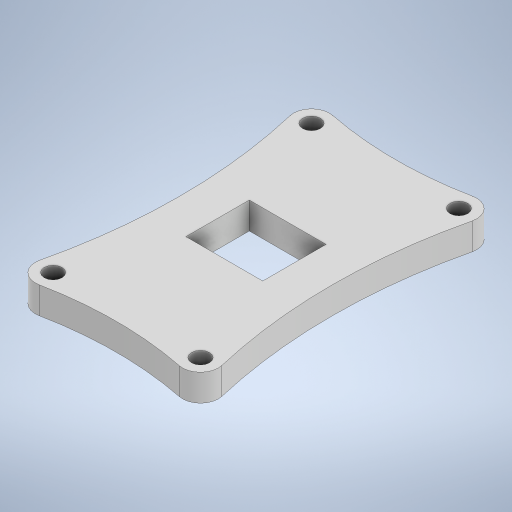
# Autodesk Inventor part: Seal_plate
Saved by Autodesk Inventor 2024.3 (Build 283343000, 343)
## iProperties
Created: 2024-11-18
Part Number: Seal_plate
Material: Generic
Document SubType Name: Modeling
Designer: magn1
Density: 1 g/cm^3
Appearance: Default
Author: magn1
Autodesk Inventor part; units mm, degrees
ref_plane "YZ Plane" through (0, 0, 0) normal (1, 0, 0) x (0, 1, 0)
ref_plane "XZ Plane" through (0, 0, 0) normal (0, 1, 0) x (-1, 0, 0)
ref_plane "XY Plane" through (0, 0, 0) normal (0, 0, 1) x (1, 0, 0)
sketch "Sketch1" plane through (0, 0, 0) normal (0, 1, 0) x (-1, 0, 0)
  line L0 (-8.25, 14.464) -> (8.25, 14.464) construction
  line L1 (8.25, 14.464) -> (8.25, -14.464) construction
  line L2 (8.25, -14.464) -> (-8.25, -14.464) construction
  line L3 (-8.25, -14.464) -> (-8.25, 14.464) construction
  line L4 (-8.25, 14.464) -> (8.25, -14.464) construction
  line L5 (8.25, 14.464) -> (-8.25, -14.464) construction
  circle A0 centre (8.25, 14.464) radius 1
  circle A1 centre (8.25, -14.464) radius 1
  circle A2 centre (-8.25, -14.464) radius 1
  circle A3 centre (-8.25, 14.464) radius 1
  line L6 (-4.3, 3.55) -> (4.3, 3.55)
  line L7 (4.3, 3.55) -> (4.3, -3.55)
  line L8 (4.3, -3.55) -> (-4.3, -3.55)
  line L9 (-4.3, -3.55) -> (-4.3, 3.55)
  line L10 (-4.3, 3.55) -> (4.3, -3.55) construction
  line L11 (4.3, 3.55) -> (-4.3, -3.55) construction
  circle A4 centre (8.25, 14.464) radius 2
  circle A5 centre (8.25, -14.464) radius 2
  circle A6 centre (-8.25, -14.464) radius 2
  circle A7 centre (-8.25, 14.464) radius 2
  arc A8 (10.1962, 14.0034) -> (10.1962, -14.0034) centre (69.3616, 0) ccw
  arc A9 (-10.1962, -14.0034) -> (-10.1962, 14.0034) centre (-69.3616, 0) ccw
  arc A10 (7.8571, -16.425) -> (-7.8571, -16.425) centre (0, -55.6458) ccw
  arc A11 (-7.8571, 16.425) -> (7.8571, 16.425) centre (0, 55.6458) ccw
  point P0 (0, 0)
  dimension "d0" = 16.5
  dimension "d1" = 28.928
  dimension "d2" = 2
  dimension "d3" = 2
  dimension "d4" = 2
  dimension "d5" = 2
  dimension "d6" = 8.6
  dimension "d7" = 7.1
  dimension "d8" = 4
  dimension "d9" = 4
  dimension "d10" = 4
  dimension "d11" = 4
  dimension "d12" = 60.8
  dimension "d13" = 60.8
  dimension "d14" = 40
  dimension "d15" = 40
  constraints: 24 end point, 16 point on circle, 12 centre point, 8 coincident, 8 tangent, 4 midpoint, 4 parallel, 2 horizontal, 2 perpendicular
  measures "d0" distance of L1.end L2.end
  measures "d1" distance of L0.end L1.end
  measures "d2" diameter of A0
  measures "d3" diameter of A1
  measures "d4" diameter of A2
  measures "d5" diameter of A3
  measures "d6" distance of L7.end L8.end
  measures "d7" distance of L6.end L7.end
  measures "d8" diameter of A4
  measures "d9" diameter of A5
  measures "d10" diameter of A6
  measures "d11" diameter of A7
  measures "d12" radius of A8
  measures "d13" radius of A9
  measures "d14" radius of A10
  measures "d15" radius of A11
extrude "Extrusion1" add sketch "Sketch1" along normal blind 3
body "Solid1"
